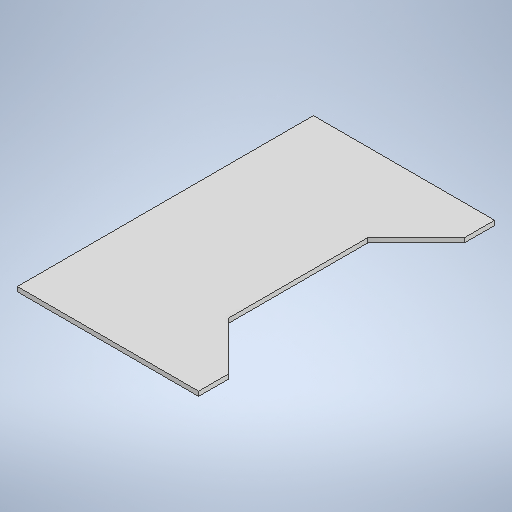
# Autodesk Inventor part: asiura_ita
Saved by Autodesk Inventor 2025.1 (Build 291241000, 241)
## iProperties
Created: 2024-09-04
Part Number: asiura_ita
Material: 一般
Document SubType Name: Modeling
Designer: right
Density: 1 g/cm^3
Appearance: 既定
Author: right
Autodesk Inventor part; units mm, degrees
ref_plane "YZ Plane" through (0, 0, 0) normal (1, 0, 0) x (0, 1, 0)
ref_plane "XZ Plane" through (0, 0, 0) normal (0, 1, 0) x (-1, 0, 0)
ref_plane "XY Plane" through (0, 0, 0) normal (0, 0, 1) x (1, 0, 0)
sketch "スケッチ1" plane through (0, 0, 0) normal (0, 1, 0) x (-1, 0, 0)
  line L0 (30, 49) -> (-30, 49)
  line L1 (-30, 49) -> (-30, -49)
  line L2 (-30, -49) -> (30, -49)
  line L3 (30, -49) -> (30, 49)
  line L4 (30, 49) -> (-30, -49) construction
  line L5 (-30, 49) -> (30, -49) construction
  line L6 (-14, -23) -> (-14, 23)
  line L7 (-14, 23) -> (-30, 39)
  line L8 (-14, -23) -> (-30, -39)
  line L9 (-30, 0) -> (30, 0) construction
  point P0 (0, 0)
  point P1 (-14, 0)
  dimension "d0" = 98
  dimension "d1" = 60
  dimension "d2" = 10
  dimension "d7" = 44
  constraints: 20 end point, 5 midpoint, 2 parallel, 2 perpendicular, 2 point on line, 1 horizontal, 1 horizontal alignment, 1 vertical, 1 other
  measures "d0" distance of L2.end L0.start
  measures "d1" distance of L1.end L2.end
  measures "d2" distance of L1.end L8.end
  measures "d7" distance between parallel lines of L3 L6
extrude "押し出し1" add sketch "スケッチ1" along normal blind 1.5 contours L3 L2 L1 L8 L6 L7 L0
